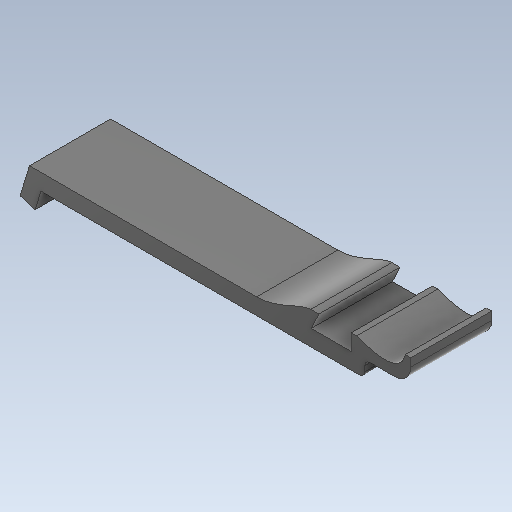
# Autodesk Inventor part: bat_lock03
Saved by Autodesk Inventor 2020 (Build 240168000, 168)
## iProperties
Created: 2023-12-19
Part Number: bat_lock03
Material: Типовые
Document SubType Name: Modeling
Designer: denis
Density: 1 g/cm^3
Appearance: По умолчанию
Author: denis
Autodesk Inventor part; units mm, degrees
ref_plane "YZ Plane" through (0, 0, 0) normal (1, 0, 0) x (0, 1, 0)
ref_plane "XZ Plane" through (0, 0, 0) normal (0, 1, 0) x (-1, 0, 0)
ref_plane "XY Plane" through (0, 0, 0) normal (0, 0, 1) x (1, 0, 0)
sketch "Эскиз1" plane through (0, 0, 0) normal (0, 0, 1) x (1, 0, 0)
  line L0 (0, 0) -> (1, 0)
  line L1 (9, 0) -> (9, -3) construction
  line L2 (9, -3) -> (3.5, -3) construction
  line L3 (0, -3) -> (0, 0)
  line L4 (0, -3) -> (-7.3989, -3)
  line L5 (-7.3989, -3) -> (-7.3989, -6) construction
  line L6 (-7.3989, -6) -> (0, -6)
  line L7 (0, -6) -> (0, -3) construction
  line L8 (0, -3) -> (2.5, -3) construction
  line L9 (2.5, -4) -> (2.5, -5)
  line L10 (1.5, -6) -> (0, -6)
  line L11 (0, -6) -> (0, -3) construction
  line L12 (-7.3989, -3) -> (-6, 0)
  line L13 (-7.3989, -3) -> (-13.5, -3) construction
  line L14 (-57.3989, -3) -> (-57.3989, -6) construction
  line L15 (-57.3989, -6) -> (-7.3989, -6)
  line L16 (-7.3989, -6) -> (-7.3989, -3) construction
  arc A0 (1.5, -6) -> (2.5, -5) centre (1.5, -5) ccw
  arc A1 (3.5, -3) -> (2.5, -4) centre (3.5, -4) ccw
  line L17 (-13.5, -3) -> (-17.5, -3) construction
  line L18 (0, 0) -> (1, 0)
  line L19 (9, 0) -> (8, 0) construction
  arc A2 (1, 0) -> (8, 0) centre (4.5, 9.3675) ccw construction
  line L20 (-57.3989, -3) -> (-59.5142, -3)
  line L21 (-59.5142, -3) -> (-62.1244, -11.5373)
  line L22 (-62.1244, -12.6534) -> (-58.474, -12.6534) construction
  line L23 (-58.474, -12.6534) -> (-58.474, -9.5163) construction
  line L24 (-58.474, -12.6534) -> (3.765, -31.6817)
  line L25 (3.765, -31.6817) -> (4.6422, -28.8128)
  line L26 (4.6422, -28.8128) -> (-58.474, -9.5163)
  line L27 (-58.474, -9.5163) -> (-58.474, -12.6534) construction
  line L28 (-57.3989, -6) -> (-57.3989, -3) construction
  line L29 (-58.474, -9.5163) -> (-57.3989, -6)
  line L30 (-13.5, -3) -> (-17.5, -3) construction
  line L31 (-17.5, -3) -> (-57.3989, -3)
  line L32 (1, 0) -> (8, 0) construction
  line L33 (8, 0) -> (9, 0) construction
  line L34 (-58.474, -12.6534) -> (-62.1244, -11.5373)
  line L35 (-62.1244, -11.5373) -> (-62.1244, -12.6534) construction
  line L36 (-6, 0) -> (-7.5, 0) construction
  line L37 (-7.5, 0) -> (-7.5, -3) construction
  line L38 (-7.5, 0) -> (-9.5, 0) construction
  line L39 (-7.5, 0) -> (-9.5, 0) construction
  line L40 (-9.5, 0) -> (-13.5, -3) construction
  line L41 (-13.5, -3) -> (-17.5, -3) construction
  spline S0 degree 3 poles (-7.5, 0) (-9.5, 0) (-13.5, -3) (-17.5, -3) knots 1 1 1 1 2 2 2 2
  line L42 (-7.5, 0) -> (-6, 0)
  line L43 (9, -3) -> (11, -3) construction
  line L44 (11, 0) -> (11, 1.5)
  line L45 (11, 1.5) -> (10.6727, 1.5)
  arc A3 (1, 0) -> (10.6727, 1.5) centre (4.5, 9.3675) ccw
  line L46 (3.5, -3) -> (8, -3)
  arc A4 (8, -3) -> (11, 0) centre (8, 0) ccw
  point P0 (2.5, -6)
  point P1 (0, -6)
  point P2 (2, -4)
  dimension "d0" = 9
  dimension "d1" = 3
  dimension "d3" = 3
  dimension "d4" = 2.5
  dimension "d5" = 3
  dimension "d6" = 50
  dimension "d9" = 1
  dimension "d10" = 1
  dimension "d11" = 4
  dimension "d13" = 3
  dimension "d14" = 1
  dimension "d15" = 1
  dimension "d16" = 10
  dimension "d17" = 3.6504
  dimension "d18" = 10
  dimension "d20" = 3
  dimension "d21" = 65.0828
  dimension "d25" = 3.677
  dimension "d26" = 66
  dimension "d27" = 90
  dimension "d28" = 107
  dimension "d29" = 65
  dimension "d30" = 6
  dimension "d31" = 3
  dimension "d32" = 1.5
  dimension "d33" = 6
  dimension "d34" = 2
  dimension "d37" = 2
  dimension "d38" = 4.5
  dimension "d39" = 3
  dimension "d40" = 2.9
  constraints: 88 end point, 17 parallel, 13 perpendicular, 12 horizontal, 10 point on circle, 9 point on line, 7 tangent, 5 centre point, 5 collinear, 3 coincident, 1 concentric, 3 other
  measures "d0" distance of L1.end L3.start
  measures "d1" distance of L1.start L1.end
  measures "d3" distance of L5.end L4.end
  measures "d4" distance of point (2.5, -6) L10.end
  measures "d5" distance of L8.end point (2.5, -6)
  measures "d6" distance of L15.end L14.end
  measures "d9" radius of A0
  measures "d10" radius of A1
  measures "d11" distance of L13.end L17.end
  measures "d13" distance between parallel lines of L13 L15
  measures "d14" distance of L0.start L0.end
  measures "d15" distance of L1.start L19.end
  measures "d16" radius of A2
  measures "d17" distance of L22.end L22.start
  measures "d18" distance of L22.start L20.end
  measures "d20" distance of L25.end L24.end
  measures "d21" distance of L22.end L24.end
  measures "d25" distance of L23.end L14.end
  measures "d26" distance of L25.end L23.end
  measures "d27" angle of L29 L26
  measures "d28" angle of L20 L21
  measures "d29" angle of L12 L4
  measures "d30" distance from line of L12.end L3
  measures "d31" distance from line of L4 L12.end
  measures "d32" distance of L12.end L36.end
  measures "d33" distance from line of L13.end L37
  measures "d34" distance of L36.end L38.end
  measures "d37" distance of L1.end L43.end
  measures "d38" distance of L43.end L44.end
  measures "d39" radius of A4
  measures "d40" distance between parallel lines of L21 L29
extrude "Выдавливание1" add sketch "Эскиз1" along normal blind 15
sketch "Эскиз3" plane through (0, 0, 15) normal (0, 0, 1) x (1, 0, 0)
  line L0 (-57.3989, -6) -> (1.5, -6) construction
  arc A0 (1.5, -6) -> (2.5, -5) centre (1.5, -5) ccw construction
  arc A1 (3.5, -3) -> (2.5, -4) centre (3.5, -4) ccw construction
  line L1 (1, 0) -> (0, 0) construction
  line L2 (0, 0) -> (0, -3) construction
  line L3 (0, -3) -> (-7.3989, -3) construction
  line L4 (-7.3989, -3) -> (-6, 0) construction
  line L5 (-6, 0) -> (-7.5, 0) construction
  line L6 (-17.5, -3) -> (-59.5142, -3) construction
  line L7 (-59.5142, -3) -> (-62.1244, -11.5373) construction
  line L8 (-62.1244, -11.5373) -> (3.765, -31.6817) construction
  line L9 (3.765, -31.6817) -> (4.6422, -28.8128) construction
  line L10 (4.6422, -28.8128) -> (-58.474, -9.5163) construction
  line L11 (-58.474, -9.5163) -> (-57.3989, -6) construction
  line L12 (4.6422, -28.8128) -> (-58.474, -9.5163) construction
  line L13 (-58.474, -9.5163) -> (-61.2472, -8.6684)
  line L14 (-58.474, -9.5163) -> (8.3891, -25.5344)
  line L15 (8.3891, -25.5344) -> (5.592, -37.2821)
  line L16 (5.592, -37.2821) -> (-67.5523, -14.3814)
  line L17 (-67.5523, -14.3814) -> (-63.6325, -8.2805)
  line L18 (-63.6325, -8.2805) -> (-61.2472, -8.6684)
  line L19 (2.5, -5) -> (2.5, -4) projected
  line L20 (3.5, -3) -> (8, -3) projected
  arc A2 (8, -3) -> (11, 0) centre (8, 0) ccw projected
  line L21 (11, 0) -> (11, 1.5) projected
  line L22 (11, 1.5) -> (10.6727, 1.5) projected
  arc A3 (1, 0) -> (10.6727, 1.5) centre (4.5, 9.3675) ccw projected
  constraints: 12 end point, 2 point on line, 1 perpendicular, 1 other
extrude "Выдавливание2" cut sketch "Эскиз3" against normal blind 25
sketch "Эскиз4" plane through (0, 0, 15) normal (0, 0, 1) x (1, 0, 0)
  line L0 (-61.2472, -8.6684) -> (-58.474, -9.5163) construction
  line L1 (-58.474, -9.5163) -> (-57.3989, -6) construction
  line L2 (-57.3989, -6) -> (1.5, -6) construction
  arc A0 (1.5, -6) -> (2.5, -5) centre (1.5, -5) ccw construction
  line L3 (2.5, -5) -> (2.5, -4) construction
  arc A1 (3.5, -3) -> (2.5, -4) centre (3.5, -4) ccw construction
  line L4 (3.5, -3) -> (8, -3) construction
  arc A2 (8, -3) -> (11, 0) centre (8, 0) ccw construction
  line L5 (11, 0) -> (11, 1.5) construction
  line L6 (11, 1.5) -> (10.6727, 1.5) construction
  arc A3 (1, 0) -> (10.6727, 1.5) centre (4.5, 9.3675) ccw construction
  line L7 (1, 0) -> (0, 0) construction
  line L8 (0, 0) -> (0, -3) construction
  line L9 (0, -3) -> (-7.3989, -3) construction
  line L10 (-7.3989, -3) -> (-6, 0) construction
  line L11 (-6, 0) -> (-7.5, 0) construction
  line L12 (-17.5, -3) -> (-59.5142, -3) construction
  line L13 (-59.5142, -3) -> (-61.2472, -8.6684) construction
  arc A4 (1, 0) -> (10.6727, 1.5) centre (4.5, 9.3675) ccw construction
  line L14 (1, 0) -> (9, -3) construction
  line L15 (9, -3) -> (10.6727, 1.5) construction
  spline S0 degree 2 poles (1, 0) (9, -3) (10.6727, 1.5) knots 1 1 1 2 2 2 construction
  line L16 (1, 0) -> (10.6727, 1.5) construction
  line L17 (11, 1.5) -> (10.6727, 1.5) projected
  line L18 (11, 1.5) -> (10, 1.5)
  line L19 (1, 0) -> (9, -3) construction
  line L20 (9, -3) -> (10, 1.5) construction
  spline S1 degree 2 poles (1, 0) (9, -3) (10, 1.5) knots 1 1 1 2 2 2
  line L21 (11, 0) -> (11, 1.5) projected
  line L22 (11, 1.5) -> (10, 0.696)
  line L23 (10, 0.696) -> (9.7197, 0.6526)
  line L24 (1, 0) -> (10, 1.5)
  dimension "d43" = 1
  constraints: 10 end point, 4 tangent, 1 coincident, 1 collinear, 1 horizontal alignment, 1 point on line, 8 other
  measures "d43" distance of L5.end L18.end
extrude "Выдавливание3" add sketch "Эскиз4" against normal up to surface (15 mm away) contours L22 L23 S1 L18 L17
extrude "Выдавливание4" cut sketch "Эскиз4" against normal up to surface (15 mm away) contours S1 L24
